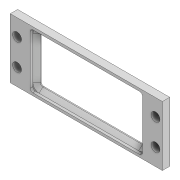
# Autodesk Inventor part: guarnizione motore
Saved by Autodesk Inventor 2022 (Build 260153000, 153)
## iProperties
Created: 2025-07-14
Part Number: guarnizione motore
Material: Generic
Document SubType Name: Modeling
Designer: 1234
Density: 1 g/cm^3
Appearance: Default
Author: 1234
Autodesk Inventor part; units mm, degrees
ref_plane "YZ Plane" through (0, 0, 0) normal (1, 0, 0) x (0, 1, 0)
ref_plane "XZ Plane" through (0, 0, 0) normal (0, 1, 0) x (-1, 0, 0)
ref_plane "XY Plane" through (0, 0, 0) normal (0, 0, 1) x (1, 0, 0)
sketch "Sketch1" plane through (0, 0, 0) normal (0, 0, 1) x (1, 0, 0)
  line L0 (0, 0) -> (-40, 0)
  line L1 (-40, 0) -> (-40, 18)
  line L2 (-40, 18) -> (0, 18)
  line L3 (0, 18) -> (0, 0)
  line L4 (1.4, 19.4) -> (-41.4, 19.4)
  line L5 (-41.4, 19.4) -> (-41.4, -1.4)
  line L6 (-41.4, -1.4) -> (1.4, -1.4)
  line L7 (1.4, -1.4) -> (1.4, 19.4)
  line L8 (-49, 20.4) -> (9, 20.4)
  line L9 (9, -2.4) -> (-49, -2.4)
  line L10 (-49, -2.4) -> (-49, 20.4)
  line L11 (-40, 9) -> (-51.8355, 9) construction
  circle A0 centre (-46.4, 14) radius 1.7
  circle A1 centre (-46.4, 4) radius 1.7
  line L12 (-46.4, 16.8208) -> (-46.4, -2.4) construction
  line L13 (-20, 18) -> (-20, -3.9948) construction
  line L14 (9, -2.4) -> (9, 20.4)
  circle A2 centre (6.4, 14) radius 1.7
  circle A3 centre (6.4, 4) radius 1.7
  dimension "d0" = 40
  dimension "d1" = 18
  dimension "d2" = 1.4
  dimension "d16" = 1
  dimension "d17" = 1
  dimension "d18" = 9
  dimension "d19" = 3.4
  dimension "d20" = 3.4
  dimension "d21" = 5
  dimension "d22" = 5
  dimension "d23" = 5
  constraints: 30 end point, 5 parallel, 4 centre point, 4 symmetric about line, 3 vertical, 2 horizontal, 2 midpoint, 2 perpendicular, 2 point on line, 5 other
  measures "d0" distance of L1.end L2.end
  measures "d1" distance of L0.end L1.end
  measures "d2" distance between parallel lines of L2 L4
  measures "d16" distance between parallel lines of L8 L4
  measures "d17" distance between parallel lines of L6 L9
  measures "d18" distance between parallel lines of L1 L10
  measures "d19" diameter of A1
  measures "d20" diameter of A0
  measures "d21" distance between parallel lines of L5 L12
  measures "d22" distance from line of L11 A0.centre
  measures "d23" distance from line of L11 A1.centre
extrude "Extrusion1" add sketch "Sketch1" along normal blind 1 contours L8 L14 L9 L10
extrude "Extrusion2" add sketch "Sketch1" against normal blind 1.8 contours L7 L6 L5 L4 | L8 L14 L9 L10
fillet "Fillet1" radius 1 8 edges at (0, 0, -0.9) (1.4, -1.4, 0.5) (-40, 0, -0.9) (-41.4, -1.4, 0.5) (-40, 18, -0.9) (-41.4, 19.4, 0.5) (1.4, 19.4, 0.5) (0, 18, -0.9)
chamfer "Chamfer2" distance 1.4 angle 45 8 edges at (0, 9, 0) (-0.2929, 0.2929, 0) (-20, 0, 0) (-39.7071, 0.2929, 0) (-40, 9, 0) (-39.7071, 17.7071, 0) (-20, 18, 0) (-0.2929, 17.7071, 0)
equation "\"d19\" = d20"
body "Solid1"
